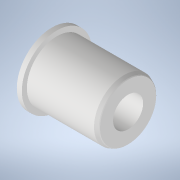
# Autodesk Inventor part: Hülse1
Saved by Autodesk Inventor 2022 (Build 260153000, 153)
## iProperties
Created: 2022-01-02
Part Number: Hülse1
Material: Generisch
Document SubType Name: Modeling
Designer: Jan
Density: 1 g/cm^3
Appearance: Vorgabe
Author: Jan
Autodesk Inventor part; units mm, degrees
ref_plane "YZ Plane" through (0, 0, 0) normal (1, 0, 0) x (0, 1, 0)
ref_plane "XZ Plane" through (0, 0, 0) normal (0, 1, 0) x (-1, 0, 0)
ref_plane "XY Plane" through (0, 0, 0) normal (0, 0, 1) x (1, 0, 0)
sketch "Skizze1" plane through (0, 0, 0) normal (0, 0, 1) x (1, 0, 0)
  line L0 (7, -3) -> (0, -3)
  line L1 (7, 3) -> (7, -3) projected
  line L2 (7, 3) -> (0, 3)
  line L3 (7, 1.8) -> (13, 1.8)
  line L4 (7, -1.8) -> (13, -1.8)
  line L5 (0, 3) -> (0, -3) projected
  line L6 (7, 0) -> (7, 3)
  line L7 (0, 3) -> (-0.1, 3)
  line L8 (-0.1, 3) -> (-0.1, 3.5)
  line L9 (-0.1, 3.5) -> (-0.6, 3.5)
  line L10 (-0.6, 3.5) -> (-0.6, 0)
  line L11 (-0.6, 0) -> (7, 0)
  point P0 (0, 0)
  point P1 (0, 0)
  dimension "d0" = 0.1
  dimension "d1" = 0.5
  dimension "d2" = 0.5
  dimension "d24" = 7.6
  dimension "d25" = 3.5
  dimension "d26" = 3
  constraints: 20 end point, 5 horizontal, 4 perpendicular, 1 coincident, 1 collinear, 1 midpoint, 7 other
  measures "d0" distance of L2.end L7.end
  measures "d1" distance of L7.end L8.end
  measures "d2" distance of L8.end L9.end
  measures "d24" distance from line of L10 L1.start
  measures "d25" distance of L10.end L9.end
  measures "d26" vertical distance of point (0, 0) L7.end
revolve "Umdrehung1" add sketch "Skizze1" angle 360 about axis through (-0.6, 0, 0) along (1, 0, 0) contours L11 L10 L9 L8 L7 L5 | L5 L2 L1 L11
sketch "Skizze3" plane through (-0.6, 0, 0) normal (-1, 0, 0) x (0, 0, 1)
  point P0 (0, 0)
chamfer "Fase1" distance 0.2 angle 45 1 edges at (7, -3, 0)
chamfer "Fase2" distance 0.2 angle 45 1 edges at (6.8, -3, 0)
hole "Bohrung2" at (-0.6, 0, 0) direction (1, 0, 0) diameter 3 end through all
chamfer "Fase3" distance 0.2 angle 45 1 edges at (-0.6, 0, -1.5)
